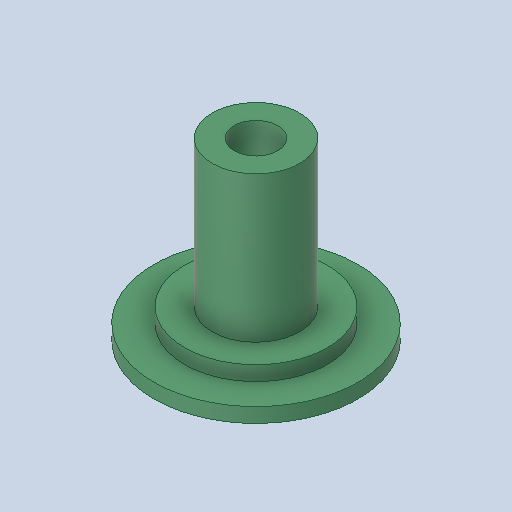
# Autodesk Inventor part: TorsOsc-202511-cell-tower
Saved by Autodesk Inventor 2026 (Build 300175050, 175E)
## iProperties
Created: 2025-12-02
Part Number: TorsOsc-202511-cell-tower
Material: Epoxy Resin
Document SubType Name: Modeling
Designer: schanen
Density: 1.14 g/cm^3
Appearance: Smooth - Dark Sea Green
Mass: 1.63522 g
Surface Area: 26.1355 cm^2
Volume: 1.24826 cm^3
Author: schanen
Autodesk Inventor part; units mm, degrees
ref_plane "YZ Plane" through (0, 0, 0) normal (1, 0, 0) x (0, 1, 0)
ref_plane "XZ Plane" through (0, 0, 0) normal (0, 1, 0) x (-1, 0, 0)
ref_plane "XY Plane" through (0, 0, 0) normal (0, 0, 1) x (1, 0, 0)
sketch "Sketch1" plane through (0, 0, 0) normal (1, 0, 0) x (0, 1, 0)
  line L0 (7, 0.625) -> (0, 0.625)
  line L1 (1, 1.45) -> (1, 3.5)
  line L2 (2, 2.45) -> (2, 1.5)
  line L3 (7, 1.5) -> (7, 0.625)
  line L4 (-1.4, 0) -> (8.4, 0) projected
  line L5 (1.5, 2.45) -> (2, 2.45)
  line L6 (1, 3.5) -> (1.5, 3.5)
  line L7 (1.5, 3.5) -> (1.5, 2.45)
  line L8 (1, 1.45) -> (0, 1.45)
  line L9 (0, 1.45) -> (0, 0.625)
  line L10 (7, 1.5) -> (2, 1.5)
  point P0 (0, 0)
  dimension "d0" = 7
  dimension "d1" = 0.625
  dimension "d8" = 2.45
  dimension "d10" = 0.5
  dimension "d11" = 0.5
  dimension "d13" = 3.5
  dimension "d16" = 1
  dimension "d31" = 1.45
  dimension "d32" = 1.5
  constraints: 20 end point, 4 horizontal, 4 perpendicular, 1 horizontal alignment, 1 vertical, 1 vertical alignment
  measures "d0" distance of L0.start L0.end
  measures "d1" distance between parallel lines of L4 L0
  measures "d8" distance between parallel lines of L4 L5
  measures "d10" distance of L1.end L6.end
  measures "d11" distance of L5.start L2.start
  measures "d13" distance between parallel lines of L4 L6
  measures "d16" distance between parallel lines of L9 L1
  measures "d31" distance from line of point (0, 0) L8
  measures "d32" distance from line of point (0, 0) L10
revolve "Revolution1" add sketch "Sketch1" angle 360 about axis through (0, -10, 0) along (0, 1, 0)
sketch "Sketch5" plane through (0, 7, 0) normal (0, 1, 0) x (1, 0, 0)
  circle A0 centre (0, 0) radius 0.75
  dimension "d28" = 1.5
  constraints: 1 centre point, 1 coincident
  measures "d28" diameter of A0
extrude "Extrusion2" cut sketch "Sketch5" against normal blind 3
body "Solid1"
